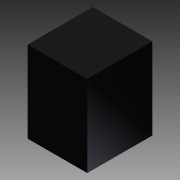
# Autodesk Inventor part: computer model
Saved by Autodesk Inventor 2012 (Build 160160000, 160)
## iProperties
Created: 2011-10-06
Part Number: computer model
Material: Default
Document SubType Name: Modeling
Designer: Antonella
Density: 1 g/cm^3
Author: Antonella
Autodesk Inventor part; units mm, degrees
ref_plane "YZ Plane" through (0, 0, 0) normal (1, 0, 0) x (0, 1, 0)
ref_plane "XZ Plane" through (0, 0, 0) normal (0, 1, 0) x (-1, 0, 0)
ref_plane "XY Plane" through (0, 0, 0) normal (0, 0, 1) x (1, 0, 0)
sketch "Sketch1" plane through (0, 0, 0) normal (0, 0, 1) x (1, 0, 0)
  line L0 (-195.58, 0) -> (195.58, 0) projected
  line L1 (0, -266.7) -> (0, 266.7) projected
  line L2 (-139.7, 190.5) -> (139.7, 190.5)
  line L3 (139.7, 190.5) -> (139.7, -190.5)
  line L4 (139.7, -190.5) -> (-139.7, -190.5)
  line L5 (-139.7, -190.5) -> (-139.7, 190.5)
  point P0 (0, 0)
  point P1 (0, 190.5)
  point P2 (-139.7, 0)
  dimension "d0" = 381
  dimension "d1" = 279.4
  constraints: 8 end point, 2 midpoint, 2 parallel, 1 horizontal, 1 horizontal alignment, 1 perpendicular, 1 vertical alignment
  measures "d0" distance of L4.end L2.start
  measures "d1" distance of L2.start L2.end
extrude "Extrusion1" add sketch "Sketch1" along normal blind 304.8
body "Solid1"
